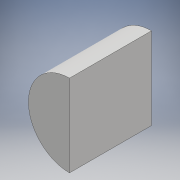
# Autodesk Inventor part: 12mm_radius_mold
Saved by Autodesk Inventor 2018 (Build 220112000, 112)
## iProperties
Created: 2018-06-11
Part Number: 12mm_radius_mold
Material: Generic
Document SubType Name: Modeling
Designer: McCormick Lab
Density: 1 g/cm^3
Appearance: Default
Author: McCormick Lab
Autodesk Inventor part; units mm, degrees
ref_plane "YZ Plane" through (0, 0, 0) normal (1, 0, 0) x (0, 1, 0)
ref_plane "XZ Plane" through (0, 0, 0) normal (0, 1, 0) x (-1, 0, 0)
ref_plane "XY Plane" through (0, 0, 0) normal (0, 0, 1) x (1, 0, 0)
sketch "Sketch1" plane through (0, 0, 0) normal (0, 1, 0) x (-1, 0, 0)
  arc A0 (0, -6) -> (0, 6) centre (0, 0) ccw
  line L0 (0, 6) -> (0, -6)
  dimension "d0" = 12
  constraints: 2 end point, 2 point on circle, 1 centre point, 1 coincident, 1 vertical
  measures "d0" diameter of A0
extrude "Extrusion1" add sketch "Sketch1" along normal blind 12
body "Solid1"
